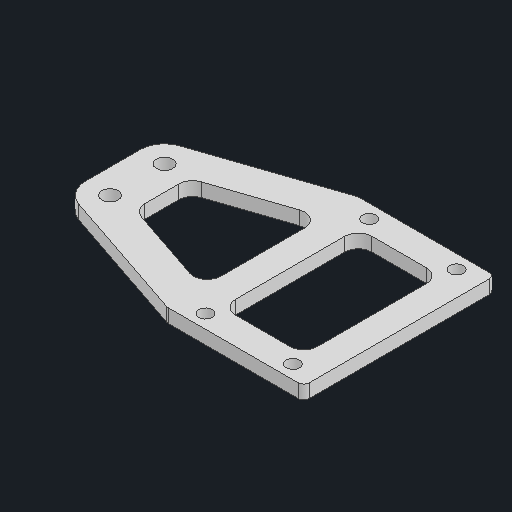
# Autodesk Inventor part: pistonMount
Saved by Autodesk Inventor 2022 (Build 260153000, 153)
## iProperties
Created: 2022-09-21
Part Number: pistonMount
Material: Generic
Document SubType Name: Modeling
Designer: Kieran Jarvis
Density: 1 g/cm^3
Appearance: Default
Author: Kieran Jarvis
Autodesk Inventor part; units mm, degrees
ref_plane "YZ Plane" through (0, 0, 0) normal (1, 0, 0) x (0, 1, 0)
ref_plane "XZ Plane" through (0, 0, 0) normal (0, 1, 0) x (-1, 0, 0)
ref_plane "XY Plane" through (0, 0, 0) normal (0, 0, 1) x (1, 0, 0)
sketch "Sketch1" plane through (0, 0, 0) normal (0, 1, 0) x (-1, 0, 0)
  circle A0 centre (0, 262.5) radius 3 construction
  circle A1 centre (0, -262.5) radius 3 construction
  line L0 (-25, -300) -> (25, -300) construction
  line L1 (25, -300) -> (25, 300) construction
  line L2 (-25, 300) -> (25, 300) construction
  line L3 (-25, -300) -> (-25, 300) construction
  circle A2 centre (71, 10) radius 3 projected
  circle A3 centre (71, -10) radius 3 projected
  arc A4 (5.8119, -39.1259) -> (-27.7565, -64.4201) centre (-3.9972, -61.0298) ccw construction
  arc A5 (-27.7597, 64.3976) -> (5.8116, 39.1072) centre (-4, 61.01) ccw construction
  line L4 (71, 10) -> (71, -10) construction
  circle A6 centre (71, -10) radius 9 construction
  circle A7 centre (71, 10) radius 9 construction
  line L5 (80, 10) -> (80, -10)
  line L6 (25, 35) -> (73.8743, 18.5287)
  line L7 (25, 35) -> (-25, 35)
  line L8 (-25, 35) -> (-25, -35)
  line L9 (-25, -35) -> (25, -35)
  line L10 (25, -35) -> (25, 35) construction
  line L11 (25, 35) -> (-25, -35) construction
  line L12 (-25, 35) -> (25, -35) construction
  line L13 (25, -35) -> (73.8743, -18.5287)
  arc A8 (80, 10) -> (73.8743, 18.5287) centre (71, 10) ccw
  arc A9 (73.8743, -18.5287) -> (80, -10) centre (71, -10) ccw
  line L14 (25, 35) -> (25, -35)
  line L15 (15, -25) -> (-15, -25)
  line L16 (-15, -25) -> (-15, 25)
  line L17 (-15, 25) -> (15, 25)
  line L18 (15, 25) -> (15, -25)
  line L19 (25, 35) -> (73.8743, 18.5287)
  line L20 (73.8743, 18.5287) -> (70.0419, 7.1571)
  line L21 (70.0419, 7.1571) -> (21.1676, 23.6284)
  line L22 (21.1676, 23.6284) -> (25, 35)
  line L23 (25, -35) -> (73.8743, -18.5287)
  line L24 (73.8743, -18.5287) -> (70.0419, -7.1571)
  line L25 (70.0419, -7.1571) -> (21.1676, -23.6284)
  line L26 (21.1676, -23.6284) -> (25, -35)
  line L27 (62, 10) -> (62, -10)
  line L28 (-25, 35) -> (-16, 35) construction
  line L29 (-16, 35) -> (-16, -35) construction
  line L30 (-16, -35) -> (-25, -35) construction
  line L31 (-25, -35) -> (-25, 35) construction
  line L32 (25, 35) -> (16, 35) construction
  line L33 (16, 35) -> (16, -35) construction
  line L34 (16, -35) -> (25, -35) construction
  line L35 (25, -35) -> (25, 35) construction
  line L36 (-25, 35) -> (25, 35) construction
  line L37 (25, 35) -> (25, 30) construction
  line L38 (25, 30) -> (-25, 30) construction
  line L39 (-25, 30) -> (-25, 35) construction
  line L40 (-25, -35) -> (25, -35) construction
  line L41 (25, -35) -> (25, -30) construction
  line L42 (25, -30) -> (-25, -30) construction
  line L43 (-25, -30) -> (-25, -35) construction
  circle A10 centre (16, 30) radius 2.5
  circle A11 centre (16, -30) radius 2.5
  circle A12 centre (-16, -30) radius 2.5
  circle A13 centre (-16, 30) radius 2.5
  point P0 (0, 0)
  point P1 (62, -9.8673)
  point P2 (25, -22.3369)
  point P3 (25, 22.3369)
  point P4 (62, 9.8673)
  dimension "d0" = 18
  dimension "d1" = 18
  dimension "d2" = 70
  dimension "d3" = 10
  dimension "d4" = 12
  dimension "d5" = 12
  dimension "d6" = 9
  dimension "d7" = 9
  dimension "d8" = 5
  dimension "d9" = 5
  dimension "d10" = 5
  dimension "d11" = 5
  dimension "d12" = 5
  dimension "d13" = 5
  constraints: 80 end point, 15 parallel, 15 point on line, 10 perpendicular, 10 point on circle, 8 centre point, 6 tangent, 5 horizontal, 4 coincident, 2 midpoint, 1 vertical, 3 other
  measures "d0" diameter of A6
  measures "d1" diameter of A7
  measures "d2" distance of L8.end L7.end
  measures "d3" distance between parallel lines of L9 L15
  measures "d4" distance of L6.end L20.end
  measures "d5" distance of L24.end L13.end
  measures "d6" distance of L29.end L30.end
  measures "d7" distance of L34.end L33.end
  measures "d8" distance of L36.end L37.end
  measures "d9" distance of L41.end L40.end
  measures "d10" diameter of A10
  measures "d11" diameter of A11
  measures "d12" diameter of A12
  measures "d13" diameter of A13
extrude "Extrusion1" add sketch "Sketch1" along normal blind 5 contours L20 A2 | L21 L14 L6 L20 A2 | A2 L20 | A2 L20 A8 L5 A9 L24 A3 L25 L27 L21 | L21 L22 L14 | L14 L25 L26 L9 L8 L7 L22 L21 | L25 A3 L24 L13 L14 | L14 L26 L25 | L24 A3 | A3 L24
fillet "Fillet1" radius 5 8 edges at (-15, 2.5, -25) (-15, 2.5, 25) (15, 2.5, 25) (15, 2.5, -25) (-25, 2.5, -22.3369) (-25, 2.5, 22.3369) (-62, 2.5, -9.8673) (-62, 2.5, 9.8673)
fillet "Fillet2" radius 2 4 edges at (25, 2.5, -35) (25, 2.5, 35) (-25, 2.5, -35) (-25, 2.5, 35)
sketch "Sketch3" plane through (0, 5, 0) normal (0, 1, 0) x (1, 0, 0)
  arc A0 (-80, -10) -> (-73.8743, -18.5287) centre (-71, -10) ccw projected
  arc A1 (-73.8743, 18.5287) -> (-80, 10) centre (-71, 10) ccw projected
  point P0 (0, 0)
  constraints: 2 coincident
hole "Hole1" at (-71, 5, 10) at (-71, 5, -10) direction (0, -1, 0) diameter 6 end through all
body "Solid1"
